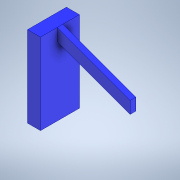
# Autodesk Inventor part: GarageSegment
Saved by Autodesk Inventor 2022.2 (Build 262287000, 287)
## iProperties
Created: 2021-11-26
Part Number: GarageSegment
Material: Wood (Walnut)
Document SubType Name: Modeling
Designer: robst
Density: 0.55 g/cm^3
Appearance: Blue - Wall Paint - Glossy
Author: robst
Autodesk Inventor part; units mm, degrees
ref_plane "YZ Plane" through (0, 0, 0) normal (1, 0, 0) x (0, 1, 0)
ref_plane "XZ Plane" through (0, 0, 0) normal (0, 1, 0) x (-1, 0, 0)
ref_plane "XY Plane" through (0, 0, 0) normal (0, 0, 1) x (1, 0, 0)
sketch "Sketch1" plane through (0, 0, 0) normal (0, 0, 1) x (1, 0, 0)
  line L0 (0, 0) -> (0, -635)
  line L1 (0, 0) -> (572.8366, -208.4955)
  line L2 (0, 0) -> (609.6, 0) construction
  line L3 (572.8366, -208.4955) -> (572.8366, -303.1009)
  line L4 (572.8366, -303.1009) -> (0, -94.6054)
  line L5 (0, 0) -> (-101.6, 0)
  line L6 (-101.6, 0) -> (-101.6, -635)
  line L7 (-101.6, -635) -> (0, -635)
  dimension "d0" = 635
  dimension "d1" = 609.6
  dimension "d2" = 20
  dimension "d3" = 88.9
  dimension "d4" = 101.6
  constraints: 16 end point, 2 horizontal, 2 perpendicular, 2 vertical, 1 equal length, 1 parallel, 1 point on line
  measures "d0" distance of L0.end L0.start
  measures "d1" distance of L0.start L1.end
  measures "d2" angle of L1 L2
  measures "d3" distance between parallel lines of L4 L1
  measures "d4" distance between parallel lines of L6 L0
extrude "Extrusion1" add sketch "Sketch1" along normal mid plane 304.8 contours L0 L7 L6 L5
extrude "Extrusion2" add sketch "Sketch1" along normal mid plane 44.45 contours L1 L3 L4 L0
body "Solid1"
